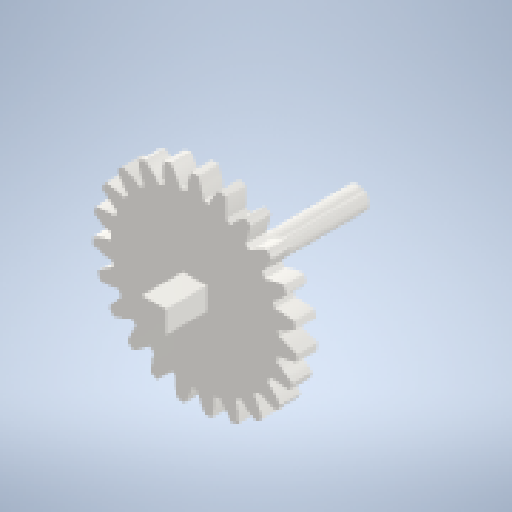
# Autodesk Inventor part: Spur Gear11_CPY
Saved by Autodesk Inventor 2023 (Build 270158000, 158)
## iProperties
Created: 2022-09-15
Part Number: Spur Gear11_CPY
Material: Steel
Document SubType Name: Modeling
Designer: simon
Categories: <?xml version="1.0" encoding="UTF-16"?> <MemberInstance><Categories><FamilyTemplate><FamilyTemplateParameter ValueType="xs:double" Id="1" ObjectReferenceKey="da_z" ObjectType="kUserParameterObject"/><FamilyTemplateParameter ValueType="xs:double" Id="2" ObjectReferenceKey="da_b" ObjectType="kUserParameterObject"/><FamilyTemplateParameter ValueType="xs:double" Id="3" ObjectReferenceKey="da_beta" ObjectType="kUserParameterObject"/><FamilyTemplateParameter ValueType="xs:double" Id="4" ObjectReferenceKey="da_da" ObjectType="kUserParameterObject"/><FamilyTemplateParameter ValueType="xs:double" Id="5" ObjectReferenceKey="da_aw" ObjectType="kUserParameterObject"/><FamilyTemplateParameter ValueType="xs:string" Id="6" ObjectReferenceKey="EAIAABAAAACIAQAAAAAAAIAAAAAAAAAA" ObjectType="83910656" SubObjectId="SurfaceGeometry"/></FamilyTemplate><ParamToTemplateMap><ParamToTemplate CategoryParameter="//CategoryParameter[@InternalName='046C89C9-8512-4d59-83FE-43B91F4F132A']" TemplateParameter="1"/><ParamToTemplate CategoryParameter="//CategoryParameter[@InternalName='2552DF32-E462-4b46-AEBF-C6C7768E72AC']" TemplateParameter="2"/><ParamToTemplate CategoryParameter="//CategoryParameter[@InternalName='C9EE641D-15FC-4fae-A226-E94C4372FDD7']" TemplateParameter="3"/><ParamToTemplate><ParamToTemplate CategoryParameter="//CategoryParameter[@InternalName='00B6519A-459B-49c7-AD84-2E56D39A5744']" ConstantValue="0.000000"/></ParamToTemplate><ParamToTemplate><ParamToTemplate CategoryParameter="//CategoryParameter[@InternalName='04B31F0E-C7A6-4894-AA32-9629BEFACF47']" ConstantValue="1.000000"/></ParamToTemplate><ParamToTemplate><ParamToTemplate CategoryParameter="//CategoryParameter[@InternalName='43CBEC2E-7847-49e7-A936-2F7889FCB2D9']" ConstantValue="0.250000"/></ParamToTemplate><ParamToTemplate><ParamToTemplate CategoryParameter="//CategoryParameter[@InternalName='B1EFC894-105D-4ebd-86BF-FA20ED196853']" ConstantValue="0.350000"/></ParamToTemplate><ParamToTemplate><ParamToTemplate CategoryParameter="//CategoryParameter[@InternalName='51175063-3D10-4879-93E8-6246FE8B403D']" ConstantValue="2060000000.000000"/></ParamToTemplate><ParamToTemplate><ParamToTemplate CategoryParameter="//CategoryParameter[@InternalName='A3A52E27-4454-46a9-B0BD-C932399B70AF']" ConstantValue="0.300000"/></ParamToTemplate><ParamToTemplate><ParamToTemplate CategoryParameter="//CategoryParameter[@InternalName='91B76062-C214-41d9-B1B9-14D2AB99603D']" ConstantValue="0.200000"/></ParamToTemplate><ParamToTemplate><ParamToTemplate CategoryParameter="//CategoryParameter[@InternalName='374E806E-8B8A-4dda-A9AA-1039D6500AD2']" ConstantValue="5.000000"/></ParamToTemplate><ParamToTemplate><ParamToTemplate CategoryParameter="//CategoryParameter[@InternalName='2D373A89-B862-43d6-8D0B-0CBF12AB9F6C']" ConstantValue="0.349066"/></ParamToTemplate><ParamToTemplate CategoryParameter="//CategoryParameter[@InternalName='37777632-D6A2-4fac-9D53-DB8ACD95C989']" TemplateParameter="4"/><ParamToTemplate CategoryParameter="//CategoryParameter[@InternalName='FD1017F1-B727-4f7e-9707-0F86F1FF9423']" TemplateParameter="5"/><ParamToTemplate><ParamToTemplate CategoryParameter="//CategoryParameter[@InternalName='9E1B4470-B2D3-4ff1-B813-535BB4CDF51A']" ConstantValue="3520000.000000"/></ParamToTemplate><ParamToTemplate><ParamToTemplate CategoryParameter="//CategoryParameter[@InternalName='F8452263-BFF6-458c-9FB1-07C4B99E95CD']" ConstantValue="11400000.000000"/></ParamToTemplate><ParamToTemplate><ParamToTemplate CategoryParameter="//CategoryParameter[@InternalName='3E3BB259-FD49-497f-8171-6EBC954A3479']" ConstantValue="2.000000"/></ParamToTemplate><ParamToTemplate CategoryParameter="//CategoryParameter[@InternalName='27C3BAF2-7550-4e4b-AE2C-0DB134B7D9B7']" TemplateParameter="6"/></ParamToTemplateMap><Category DisplayName="Gear" InternalName="DC85795E-93AB-48d5-8EEE-5A27447B64BD" Mnemonic="Gear"><CategoryParameter DisplayName="z" InternalName="046C89C9-8512-4d59-83FE-43B91F4F132A" Mnemonic="z"/><CategoryParameter DisplayName="b" InternalName="2552DF32-E462-4b46-AEBF-C6C7768E72AC" Mnemonic="b"/><CategoryParameter DisplayName="||b|" InternalName="C9EE641D-15FC-4fae-A226-E94C4372FDD7" Mnemonic="beta"/><CategoryParameter DisplayName="x" InternalName="00B6519A-459B-49c7-AD84-2E56D39A5744" Mnemonic="x"/><CategoryParameter DisplayName="a*" InternalName="04B31F0E-C7A6-4894-AA32-9629BEFACF47" Mnemonic="a"/><CategoryParameter DisplayName="c*" InternalName="43CBEC2E-7847-49e7-A936-2F7889FCB2D9" Mnemonic="c"/><CategoryParameter DisplayName="r|.f|*" InternalName="B1EFC894-105D-4ebd-86BF-FA20ED196853" Mnemonic="rf"/><CategoryParameter DisplayName="E" InternalName="51175063-3D10-4879-93E8-6246FE8B403D" Mnemonic="E"/><CategoryParameter DisplayName="||m|" InternalName="A3A52E27-4454-46a9-B0BD-C932399B70AF" Mnemonic="mi"/><Category DisplayName="SpurGear" InternalName="26C5A22E-A91E-4dfd-A3B3-23CCAFAE1764" Mnemonic="SpurGear"><CategoryParameter DisplayName="m" InternalName="91B76062-C214-41d9-B1B9-14D2AB99603D" Mnemonic="m"/><CategoryParameter DisplayName="P" InternalName="374E806E-8B8A-4dda-A9AA-1039D6500AD2" Mnemonic="PP"/><CategoryParameter DisplayName="||a|" InternalName="2D373A89-B862-43d6-8D0B-0CBF12AB9F6C" Mnemonic="alpha"/><CategoryParameter DisplayName="d|.a|" InternalName="37777632-D6A2-4fac-9D53-DB8ACD95C989" Mnemonic="da"/><CategoryParameter DisplayName="a|.w|" InternalName="FD1017F1-B727-4f7e-9707-0F86F1FF9423" Mnemonic="aw"/><CategoryParameter DisplayName="||s||.Flim|" InternalName="9E1B4470-B2D3-4ff1-B813-535BB4CDF51A" Mnemonic="sFlim"/><CategoryParameter DisplayName="||s||.Hlim|" InternalName="F8452263-BFF6-458c-9FB1-07C4B99E95CD" Mnemonic="sHlim"/><CategoryParameter DisplayName="type" InternalName="3E3BB259-FD49-497f-8171-6EBC954A3479" Mnemonic="type"/><CategoryParameter DisplayName="PitchDiameter" InternalName="27C3BAF2-7550-4e4b-AE2C-0DB134B7D9B7" Mnemonic="IDS_PITCHDIAM"/></Category></Category></Categories></MemberInstance>
Density: 1 g/cm^3
Appearance: Plate
CustomPartVersion: 1
Author: simon
Autodesk Inventor part; units mm, degrees
ref_plane "YZ Plane" through (0, 0, 0) normal (1, 0, 0) x (0, 1, 0)
ref_plane "XZ Plane" through (0, 0, 0) normal (0, 1, 0) x (-1, 0, 0)
ref_plane "XY Plane" through (0, 0, 0) normal (0, 0, 1) x (1, 0, 0)
sketch "Sketch1" plane through (0, 0, 0) normal (0, 0, 1) x (1, 0, 0)
  circle A0 centre (0, 0) radius 25
  dimension "d0" = 50
  constraints: 1 centre point
  measures "d0" diameter of A0
extrude "Extrusion1" add sketch "Sketch1" along normal blind 5
ref_plane "Work Plane2" through (0, 0, 2.5) normal (0, 0, 1) x (1, 0, 0)
sketch "Sketch2" plane through (0, 0, 0) normal (0, 0, -1) x (-1, 0, 0)
  circle A0 centre (0, 0) radius 25 projected
  circle A1 centre (0, 0) radius 23
  dimension "d3" = 46
  constraints: 1 centre point, 1 coincident
  measures "d3" diameter of A1
surface extrude "Pitch Diameter" sketch "Sketch2" against normal through all shown no curves A1
ref_plane "Work Plane8" through (0, 0, 0) normal (0.9906859, 0.1361666, 0) x (0, 0, 1)
ref_plane "Work Plane9" through (0, 0, 0) normal (1, 0, 0) x (0, 1, 0)
spur gear teeth "Spur Gear" teeth 23 pitch diameter 46 tip diameter 50 root diameter 41 face width 20 start plane through (0, 0, 0) normal (0, 0, -1) x (-1, 0, 0)
sketch "Sketch3" plane through (0, 0, 0) normal (0, 0, -1) x (-1, 0, 0)
  arc A0 (7.5205, 19.0707) -> (7.5629, 23.8286) centre (-10.0684, 21.6064) ccw projected
  arc A1 (7.5629, 23.8286) -> (5.9191, 24.2892) centre (0, 0) ccw projected
  arc A2 (5.9191, 24.2892) -> (3.4832, 20.2019) centre (19.829, 13.2296) ccw projected
  arc A3 (3.4832, 20.2019) -> (2.0964, 20.3925) centre (0, 0) ccw projected
  arc A4 (2.0964, 20.3925) -> (0.8535, 24.9854) centre (-15.5244, 18.0888) ccw projected
  arc A5 (0.8535, 24.9854) -> (-0.8535, 24.9854) centre (0, 0) ccw projected
  arc A6 (-0.8535, 24.9854) -> (-2.0964, 20.3925) centre (15.5244, 18.0888) ccw projected
  arc A7 (-2.0964, 20.3925) -> (-3.4832, 20.2019) centre (0, 0) ccw projected
  arc A8 (-3.4832, 20.2019) -> (-5.9191, 24.2892) centre (-19.829, 13.2296) ccw projected
  arc A9 (-5.9191, 24.2892) -> (-7.5629, 23.8286) centre (0, 0) ccw projected
  arc A10 (-7.5629, 23.8286) -> (-7.5205, 19.0707) centre (10.0684, 21.6064) ccw projected
  arc A11 (-7.5205, 19.0707) -> (-8.8044, 18.513) centre (0, 0) ccw projected
  arc A12 (-8.8044, 18.513) -> (-12.2528, 21.7915) centre (-22.663, 7.3892) ccw projected
  arc A13 (-12.2528, 21.7915) -> (-13.7113, 20.9046) centre (0, 0) ccw projected
  arc A14 (-13.7113, 20.9046) -> (-12.3868, 16.3345) centre (3.8657, 23.5216) ccw projected
  arc A15 (-12.3868, 16.3345) -> (-13.4727, 15.4511) centre (0, 0) ccw projected
  arc A16 (-13.4727, 15.4511) -> (-17.6777, 17.6777) centre (-23.8161, 1.0008) ccw projected
  arc A17 (-17.6777, 17.6777) -> (-18.8428, 16.4301) centre (0, 0) ccw projected
  arc A18 (-18.8428, 16.4301) -> (-16.3345, 12.3868) centre (-2.6237, 23.6923) ccw projected
  arc A19 (-16.3345, 12.3868) -> (-17.1417, 11.2433) centre (0, 0) ccw projected
  arc A20 (-17.1417, 11.2433) -> (-21.7915, 12.2528) centre (-23.203, -5.4619) ccw projected
  arc A21 (-21.7915, 12.2528) -> (-22.5769, 10.7371) centre (0, 0) ccw projected
  arc A22 (-22.5769, 10.7371) -> (-19.0707, 7.5205) centre (-8.9185, 22.1059) ccw projected
  arc A23 (-19.0707, 7.5205) -> (-19.5395, 6.2015) centre (0, 0) ccw projected
  arc A24 (-19.5395, 6.2015) -> (-24.2892, 5.9191) centre (-20.869, -11.5194) ccw projected
  arc A25 (-24.2892, 5.9191) -> (-24.6365, 4.2478) centre (0, 0) ccw projected
  arc A26 (-24.6365, 4.2478) -> (-20.3925, 2.0964) centre (-14.5519, 18.88) ccw projected
  arc A27 (-20.3925, 2.0964) -> (-20.488, 0.6999) centre (0, 0) ccw projected
  arc A28 (-20.488, 0.6999) -> (-24.9854, -0.8535) centre (-16.9872, -16.7226) ccw projected
  arc A29 (-24.9854, -0.8535) -> (-24.8689, -2.5566) centre (0, 0) ccw projected
  arc A30 (-24.8689, -2.5566) -> (-20.2019, -3.4832) centre (-19.106, 14.2538) ccw projected
  arc A31 (-20.2019, -3.4832) -> (-19.9171, -4.8537) centre (0, 0) ccw projected
  arc A32 (-19.9171, -4.8537) -> (-23.8286, -7.5629) centre (-11.8455, -20.6856) ccw projected
  arc A33 (-23.8286, -7.5629) -> (-23.257, -9.1714) centre (0, 0) ccw projected
  arc A34 (-23.257, -9.1714) -> (-18.513, -8.8044) centre (-22.2431, 8.5705) ccw projected
  arc A35 (-18.513, -8.8044) -> (-17.869, -10.0473) centre (0, 0) ccw projected
  arc A36 (-17.869, -10.0473) -> (-20.9046, -13.7113) centre (-5.8254, -23.1144) ccw projected
  arc A37 (-20.9046, -13.7113) -> (-19.9201, -15.1059) centre (0, 0) ccw projected
  arc A38 (-19.9201, -15.1059) -> (-15.4511, -13.4727) centre (-23.7306, 2.2515) ccw projected
  arc A39 (-15.4511, -13.4727) -> (-14.4957, -14.4957) centre (0, 0) ccw projected
  arc A40 (-14.4957, -14.4957) -> (-16.4301, -18.8428) centre (0.6268, -23.8289) ccw projected
  arc A41 (-16.4301, -18.8428) -> (-15.1059, -19.9201) centre (0, 0) ccw projected
  arc A42 (-15.1059, -19.9201) -> (-11.2433, -17.1417) centre (-23.4581, -4.2344) ccw projected
  arc A43 (-11.2433, -17.1417) -> (-10.0473, -17.869) centre (0, 0) ccw projected
  arc A44 (-10.0473, -17.869) -> (-10.7371, -22.5769) centre (7.0326, -22.7762) ccw projected
  arc A45 (-10.7371, -22.5769) -> (-9.1714, -23.257) centre (0, 0) ccw projected
  arc A46 (-9.1714, -23.257) -> (-6.2015, -19.5395) centre (-21.4457, -10.4063) ccw projected
  arc A47 (-6.2015, -19.5395) -> (-4.8537, -19.9171) centre (0, 0) ccw projected
  arc A48 (-4.8537, -19.9171) -> (-4.2478, -24.6365) centre (12.9167, -20.0342) ccw projected
  arc A49 (-4.2478, -24.6365) -> (-2.5566, -24.8689) centre (0, 0) ccw projected
  arc A50 (-2.5566, -24.8689) -> (-0.6999, -20.488) centre (-17.8429, -15.8064) ccw projected
  arc A51 (-0.6999, -20.488) -> (0.6999, -20.488) centre (0, 0) ccw projected
  arc A52 (0.6999, -20.488) -> (2.5566, -24.8689) centre (17.8429, -15.8064) ccw projected
  arc A53 (2.5566, -24.8689) -> (4.2478, -24.6365) centre (0, 0) ccw projected
  arc A54 (4.2478, -24.6365) -> (4.8537, -19.9171) centre (-12.9167, -20.0342) ccw projected
  arc A55 (4.8537, -19.9171) -> (6.2015, -19.5395) centre (0, 0) ccw projected
  arc A56 (6.2015, -19.5395) -> (9.1714, -23.257) centre (21.4457, -10.4063) ccw projected
  arc A57 (9.1714, -23.257) -> (10.7371, -22.5769) centre (0, 0) ccw projected
  arc A58 (10.7371, -22.5769) -> (10.0473, -17.869) centre (-7.0326, -22.7762) ccw projected
  arc A59 (10.0473, -17.869) -> (11.2433, -17.1417) centre (0, 0) ccw projected
  arc A60 (11.2433, -17.1417) -> (15.1059, -19.9201) centre (23.4581, -4.2344) ccw projected
  arc A61 (15.1059, -19.9201) -> (16.4301, -18.8428) centre (0, 0) ccw projected
  arc A62 (16.4301, -18.8428) -> (14.4957, -14.4957) centre (-0.6268, -23.8289) ccw projected
  arc A63 (14.4957, -14.4957) -> (15.4511, -13.4727) centre (0, 0) ccw projected
  arc A64 (15.4511, -13.4727) -> (19.9201, -15.1059) centre (23.7306, 2.2515) ccw projected
  arc A65 (19.9201, -15.1059) -> (20.9046, -13.7113) centre (0, 0) ccw projected
  arc A66 (20.9046, -13.7113) -> (17.869, -10.0473) centre (5.8254, -23.1144) ccw projected
  arc A67 (17.869, -10.0473) -> (18.513, -8.8044) centre (0, 0) ccw projected
  arc A68 (18.513, -8.8044) -> (23.257, -9.1714) centre (22.2431, 8.5705) ccw projected
  arc A69 (23.257, -9.1714) -> (23.8286, -7.5629) centre (0, 0) ccw projected
  arc A70 (23.8286, -7.5629) -> (19.9171, -4.8537) centre (11.8455, -20.6856) ccw projected
  arc A71 (19.9171, -4.8537) -> (20.2019, -3.4832) centre (0, 0) ccw projected
  arc A72 (20.2019, -3.4832) -> (24.8689, -2.5566) centre (19.106, 14.2538) ccw projected
  arc A73 (24.8689, -2.5566) -> (24.9854, -0.8535) centre (0, 0) ccw projected
  arc A74 (24.9854, -0.8535) -> (20.488, 0.6999) centre (16.9872, -16.7226) ccw projected
  arc A75 (20.488, 0.6999) -> (20.3925, 2.0964) centre (0, 0) ccw projected
  arc A76 (20.3925, 2.0964) -> (24.6365, 4.2478) centre (14.5519, 18.88) ccw projected
  arc A77 (24.6365, 4.2478) -> (24.2892, 5.9191) centre (0, 0) ccw projected
  arc A78 (24.2892, 5.9191) -> (19.5395, 6.2015) centre (20.869, -11.5194) ccw projected
  arc A79 (19.5395, 6.2015) -> (19.0707, 7.5205) centre (0, 0) ccw projected
  arc A80 (19.0707, 7.5205) -> (22.5769, 10.7371) centre (8.9185, 22.1059) ccw projected
  arc A81 (22.5769, 10.7371) -> (21.7915, 12.2528) centre (0, 0) ccw projected
  arc A82 (21.7915, 12.2528) -> (17.1417, 11.2433) centre (23.203, -5.4619) ccw projected
  arc A83 (17.1417, 11.2433) -> (16.3345, 12.3868) centre (0, 0) ccw projected
  arc A84 (16.3345, 12.3868) -> (18.8428, 16.4301) centre (2.6237, 23.6923) ccw projected
  arc A85 (18.8428, 16.4301) -> (17.6777, 17.6777) centre (0, 0) ccw projected
  arc A86 (17.6777, 17.6777) -> (13.4727, 15.4511) centre (23.8161, 1.0008) ccw projected
  arc A87 (13.4727, 15.4511) -> (12.3868, 16.3345) centre (0, 0) ccw projected
  arc A88 (12.3868, 16.3345) -> (13.7113, 20.9046) centre (-3.8657, 23.5216) ccw projected
  arc A89 (13.7113, 20.9046) -> (12.2528, 21.7915) centre (0, 0) ccw projected
  arc A90 (12.2528, 21.7915) -> (8.8044, 18.513) centre (22.663, 7.3892) ccw projected
  arc A91 (8.8044, 18.513) -> (7.5205, 19.0707) centre (0, 0) ccw projected
  circle A92 centre (0, 0) radius 2.75
  dimension "d49" = 5.5
  constraints: 1 centre point, 1 coincident
  measures "d49" diameter of A92
extrude "Extrusion2" add sketch "Sketch3" along normal blind 35 contours A92
sketch "Sketch4" plane through (0, 0, 5) normal (0, 0, 1) x (1, 0, 0)
  circle A0 centre (0, 0) radius 4
  line L0 (-2.9047, 2.75) -> (2.9047, 2.75)
  line L1 (2.9047, 2.75) -> (2.9047, -2.75)
  line L2 (2.9047, -2.75) -> (-2.9047, -2.75)
  line L3 (-2.9047, -2.75) -> (-2.9047, 2.75)
  line L4 (-2.9047, 2.75) -> (2.9047, -2.75) construction
  line L5 (2.9047, 2.75) -> (-2.9047, -2.75) construction
  dimension "d52" = 8
  constraints: 12 end point, 2 midpoint, 2 parallel, 1 coincident, 1 horizontal, 1 perpendicular, 3 other
extrude "Extrusion3" add sketch "Sketch4" along normal blind 10 contours L1 L2 L3 L0
equation "\"d0\" = da_da"
equation "\"d3\" = da_d"
equation "\"da_da\" = 50"
equation "\"da_d\" = 46"
body "Solid1"
body "Srf1"
